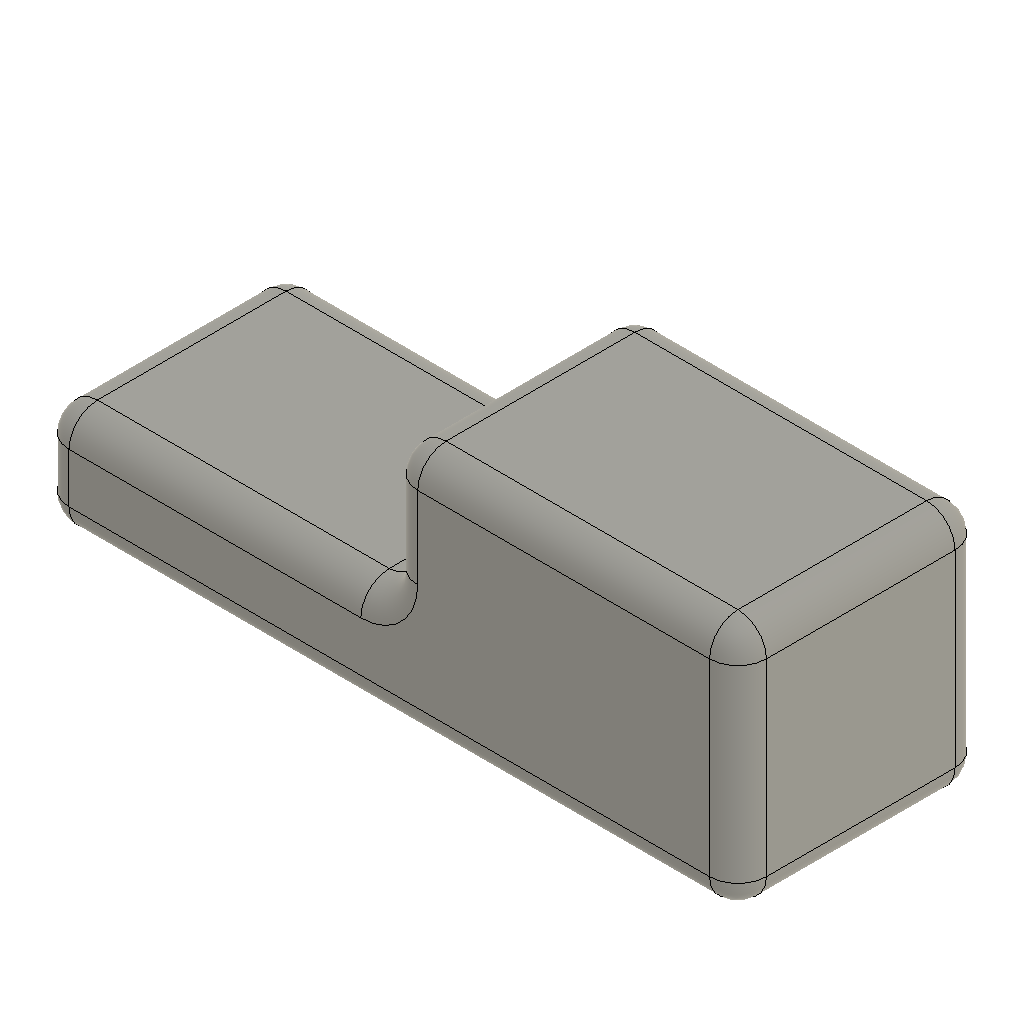
Connector_Special (Autodesk Fusion 360 design; units mm, degrees)
Autodesk Fusion 360 part; units mm, degrees
sketch "Sketch1" plane through (0, 0, 0) normal (1, 0, 0) x (0, 1, 0)
  line L0 (1.725, -1.725) -> (-1.725, -1.725)
  line L1 (-1.725, -1.725) -> (-1.725, 1.725)
  line L2 (-1.725, 1.725) -> (1.725, 1.725)
  line L3 (1.725, 1.725) -> (1.725, -1.725)
  line L4 (1.725, -1.725) -> (-1.725, 1.725) construction
  line L5 (-1.725, -1.725) -> (1.725, 1.725) construction
  line L6 (-1.725, -1.725) -> (1.725, -1.725)
  line L7 (1.725, -1.725) -> (1.725, -0.225)
  line L8 (1.725, -0.225) -> (-1.725, -0.225)
  line L9 (-1.725, -0.225) -> (-1.725, -1.725)
  dimension "d1" = 3.45
  dimension "d2" = 3.45
  dimension "d7" = 1.5
  constraint horizontal L0
  constraint perpendicular L0 L1
  constraint parallel L0 L2
  constraint parallel L1 L3
  constraint coincident L4 origin
  constraint coincident L5 origin
  constraint horizontal L6
  constraint vertical L7
  constraint horizontal L8
  constraint vertical L9
  constraint coincident L3 L7.end
  measures "d1" distance of L1.end L2.end
  measures "d2" distance of L0.end L1.end
  measures "d7" distance of L0.end L8.end
extrude "Extrude1" add sketch "Sketch1" against normal blind 4.9 contours L0 L1 L3 L6 L7 L8 L9
extrude "Extrude3" add sketch "Sketch1" along normal blind 4.9
fillet "Fillet1" radius 0.4 10 edges at (-2.45, -1.725, -0.225) (-2.45, 1.725, -0.225) (0, 0, -0.225) (0, 0, 1.725) (0, -1.725, 0.75) (0, -1.725, -1.725) (2.45, -1.725, 1.725) (2.45, 1.725, 1.725) (0, 1.725, -1.725) (0, 1.725, 0.75) 2 faces at (4.9, -0.575, 0.575) (-4.9, 0.575, -1.225)
equation "d2 = d1"
named bodies: "Connector_Special"
